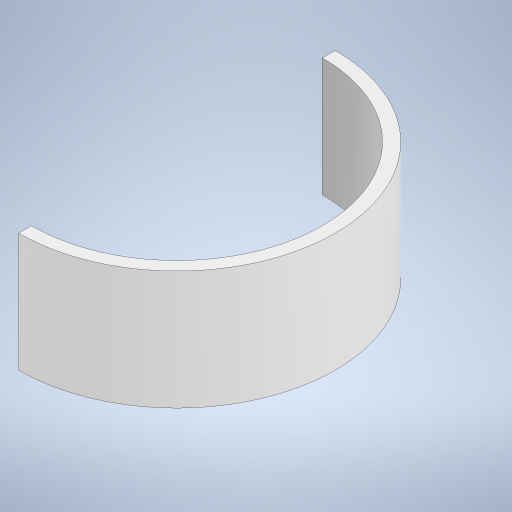
# Autodesk Inventor part: Parte media R2D2
Saved by Autodesk Inventor 2023 (Build 270158000, 158)
## iProperties
Created: 2022-10-09
Part Number: Parte media R2D2
Material: Generic
Document SubType Name: Modeling
Designer: User
Density: 1 g/cm^3
Appearance: Default
Author: User
## iProperties of the stored document Parte media R2D2_3DPrint.ipt
Created: 2022-10-18
Part Number: Parte media R2D2_3DPrint
Material: Generic
Document SubType Name: Modeling
Designer: User
Density: 1 g/cm^3
Appearance: Default
Author: User
Autodesk Inventor part; units mm, degrees
ref_plane "YZ Plane" through (0, 0, 0) normal (1, 0, 0) x (0, 1, 0)
ref_plane "XZ Plane" through (0, 0, 0) normal (0, 1, 0) x (-1, 0, 0)
ref_plane "XY Plane" through (0, 0, 0) normal (0, 0, 1) x (1, 0, 0)
sketch "Sketch1" plane through (0, 0, 0) normal (0, 1, 0) x (-1, 0, 0)
  arc A0 (0, 80) -> (0, -80) centre (0, 0) ccw
  arc A1 (0, 77) -> (0, -77) centre (0, 0) ccw
  line L0 (0, -80) -> (0, 80)
  dimension "d0" = 160
  dimension "d1" = 3
  constraints: 4 point on circle, 2 centre point, 2 coincident, 2 end point, 2 point on line, 1 vertical
  measures "d0" diameter of A0
  measures "d1" radial gap between concentric circles of A0 A1
extrude "Extrusion1" add sketch "Sketch1" along normal blind 60
sketch "Sketch3" plane through (0, 60, 0) normal (0, 1, 0) x (1, 0, 0)
  arc A0 (0, -73.5) -> (0, 73.5) centre (0, 0) ccw
  arc A1 (0, -80) -> (0, 80) centre (0, 0) ccw projected
  line L0 (0, 80) -> (0, -80) projected
  line L1 (0, 73.5) -> (0, -73.5)
  dimension "d11" = 147
  constraints: 2 end point, 2 point on circle, 2 point on line, 1 centre point, 1 coincident
  measures "d11" diameter of A0
extrude "Extrusion4" cut sketch "Sketch3" against normal blind 60 contours L0 A0
body "Solid1"
